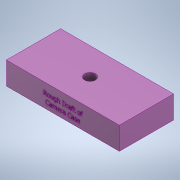
# Autodesk Inventor part: RaspberryPiCameraCase
Saved by Autodesk Inventor 2020.1 (Build 241239000, 239)
## iProperties
Created: 2019-10-02
Part Number: RaspberryPiCameraCase
Material: PC/ABS Plastic
Document SubType Name: Modeling
Designer: steele
Density: 0.357273 g/cm^3
Appearance: Smooth - Purple
Author: steele
Autodesk Inventor part; units mm, degrees
ref_plane "YZ Plane" through (0, 0, 0) normal (1, 0, 0) x (0, 1, 0)
ref_plane "XZ Plane" through (0, 0, 0) normal (0, 1, 0) x (-1, 0, 0)
ref_plane "XY Plane" through (0, 0, 0) normal (0, 0, 1) x (1, 0, 0)
sketch "Sketch1" plane through (0, 0, 0) normal (0, 1, 0) x (-1, 0, 0)
  line L0 (39.6875, 19.05) -> (-39.6875, 19.05)
  line L1 (-39.6875, 19.05) -> (-39.6875, -19.05)
  line L2 (-39.6875, -19.05) -> (39.6875, -19.05)
  line L3 (39.6875, -19.05) -> (39.6875, 19.05)
  line L4 (39.6875, 19.05) -> (-39.6875, -19.05) construction
  line L5 (-39.6875, 19.05) -> (39.6875, -19.05) construction
  point P0 (0, 0)
  dimension "d0" = 79.375
  dimension "d1" = 38.1
  constraints: 12 end point, 2 midpoint, 2 parallel, 1 horizontal, 1 perpendicular
  measures "d0" distance of L1.end L2.end
  measures "d1" distance of L2.end L0.start
extrude "Extrusion1" add sketch "Sketch1" against normal blind 15.875
sketch "Sketch2" plane through (0, 0, 0) normal (0, 1, 0) x (1, 0, 0)
  circle A0 centre (0, 0) radius 3.81
  dimension "d4" = 7.62
  constraints: 1 centre point, 1 coincident
  measures "d4" diameter of A0
extrude "Extrusion2" cut sketch "Sketch2" against normal through all
sketch "Sketch3" plane through (0, -15.875, 0) normal (0, -1, 0) x (1, 0, 0)
  point P0 (0, 0)
sketch "Sketch4" plane through (-39.6875, 0, 19.05) normal (0, 0, 1) x (1, 0, 0)
  line L0 (0, 0) -> (0, -15.875) construction
  line L1 (0, -7.9375) -> (79.375, -7.9375) construction
  line L2 (79.375, 0) -> (79.375, -15.875) construction
  line L3 (28.6181, -7.9375) -> (28.092, -7.9375)
  line L4 (28.092, -7.9375) -> (27.1287, -6.7247)
  line L5 (27.1287, -6.7247) -> (26.6643, -6.7247)
  line L6 (26.6643, -6.7247) -> (26.6643, -7.9375)
  line L7 (26.6643, -7.9375) -> (26.2593, -7.9375)
  line L8 (26.2593, -7.9375) -> (26.2593, -4.8895)
  line L9 (26.2593, -4.8895) -> (27.0447, -4.8895)
  spline S0 degree 2 poles (27.0447, -4.8895) (27.3065, -4.8895) (27.6598, -4.9463) (27.8203, -5.0501) knots 0 0 0 1 2 2 2
  spline S1 degree 2 poles (27.8203, -5.0501) (27.9809, -5.1538) (28.1661, -5.4774) (28.1661, -5.717) knots 0 0 0 1 2 2 2
  spline S2 degree 2 poles (28.1661, -5.717) (28.1661, -6.0504) (27.8252, -6.5024) (27.5338, -6.6111) knots 0 0 0 1 2 2 2
  line L10 (27.5338, -6.6111) -> (28.6181, -7.9375)
  spline S3 degree 2 poles (27.7437, -5.7491) (27.7437, -5.6157) (27.6499, -5.4107) (27.5511, -5.344) knots 0 0 0 1 2 2 2
  spline S4 degree 2 poles (27.5511, -5.344) (27.4646, -5.2872) (27.2349, -5.2402) (27.067, -5.2402) knots 0 0 0 1 2 2 2
  line L11 (27.067, -5.2402) -> (26.6643, -5.2402)
  line L12 (26.6643, -5.2402) -> (26.6643, -6.3863)
  line L13 (26.6643, -6.3863) -> (27.02, -6.3863)
  spline S5 degree 2 poles (27.02, -6.3863) (27.1954, -6.3863) (27.4745, -6.3246) (27.5708, -6.2282) knots 0 0 0 1 2 2 2
  spline S6 degree 2 poles (27.5708, -6.2282) (27.6598, -6.1443) (27.7437, -5.9071) (27.7437, -5.7491) knots 0 0 0 1 2 2 2
  spline S7 degree 2 poles (30.7102, -6.7939) (30.7102, -7.3719) (30.1545, -8.0017) (29.6901, -8.0017) knots 0 0 0 1 2 2 2
  spline S8 degree 2 poles (29.6901, -8.0017) (29.2134, -8.0017) (28.6675, -7.3521) (28.6675, -6.7939) knots 0 0 0 1 2 2 2
  spline S9 degree 2 poles (28.6675, -6.7939) (28.6675, -6.2208) (29.2307, -5.586) (29.6901, -5.586) knots 0 0 0 1 2 2 2
  spline S10 degree 2 poles (29.6901, -5.586) (30.1545, -5.586) (30.7102, -6.2184) (30.7102, -6.7939) knots 0 0 0 1 2 2 2
  spline S11 degree 2 poles (30.3126, -6.7939) (30.3126, -6.3493) (29.989, -5.917) (29.6901, -5.917) knots 0 0 0 1 2 2 2
  spline S12 degree 2 poles (29.6901, -5.917) (29.3912, -5.917) (29.0652, -6.3493) (29.0652, -6.7939) knots 0 0 0 1 2 2 2
  spline S13 degree 2 poles (29.0652, -6.7939) (29.0652, -7.2261) (29.3912, -7.6707) (29.6901, -7.6707) knots 0 0 0 1 2 2 2
  spline S14 degree 2 poles (29.6901, -7.6707) (29.9865, -7.6707) (30.3126, -7.2335) (30.3126, -6.7939) knots 0 0 0 1 2 2 2
  line L14 (32.8838, -7.9375) -> (32.4985, -7.9375)
  line L15 (32.4985, -7.9375) -> (32.4985, -7.6856)
  spline S15 degree 2 poles (32.4985, -7.6856) (32.3207, -7.8412) (32.002, -8.0017) (31.8044, -8.0017) knots 0 0 0 1 2 2 2
  spline S16 degree 2 poles (31.8044, -8.0017) (31.6562, -8.0017) (31.392, -7.9029) (31.2956, -7.7967) knots 0 0 0 1 2 2 2
  spline S17 degree 2 poles (31.2956, -7.7967) (31.1968, -7.6905) (31.0881, -7.3669) (31.0881, -7.1347) knots 0 0 0 1 2 2 2
  line L16 (31.0881, -7.1347) -> (31.0881, -5.6503)
  line L17 (31.0881, -5.6503) -> (31.4735, -5.6503)
  line L18 (31.4735, -5.6503) -> (31.4735, -6.9544)
  spline S18 degree 2 poles (31.4735, -6.9544) (31.4735, -7.1372) (31.5006, -7.3768) (31.5476, -7.4657) knots 0 0 0 1 2 2 2
  spline S19 degree 2 poles (31.5476, -7.4657) (31.5945, -7.5546) (31.755, -7.6362) (31.9057, -7.6362) knots 0 0 0 1 2 2 2
  spline S20 degree 2 poles (31.9057, -7.6362) (32.0465, -7.6362) (32.3651, -7.4756) (32.4985, -7.3595) knots 0 0 0 1 2 2 2
  line L19 (32.4985, -7.3595) -> (32.4985, -5.6503)
  line L20 (32.4985, -5.6503) -> (32.8838, -5.6503)
  line L21 (32.8838, -5.6503) -> (32.8838, -7.9375)
  spline S21 degree 2 poles (33.5236, -8.3031) (33.5631, -8.3204) (33.7138, -8.3747) (33.8101, -8.3969) knots 0 0 0 1 2 2 2
  spline S22 degree 2 poles (33.8101, -8.3969) (33.9163, -8.4241) (34.0966, -8.4562) (34.2028, -8.4562) knots 0 0 0 1 2 2 2
  spline S23 degree 2 poles (34.2028, -8.4562) (34.3807, -8.4562) (34.6277, -8.3623) (34.6968, -8.2784) knots 0 0 0 1 2 2 2
  spline S24 degree 2 poles (34.6968, -8.2784) (34.7635, -8.1944) (34.8154, -7.9746) (34.8154, -7.8338) knots 0 0 0 1 2 2 2
  line L22 (34.8154, -7.8338) -> (34.8154, -7.6337)
  spline S25 degree 2 poles (34.8154, -7.6337) (34.6598, -7.7695) (34.3609, -7.898) (34.1361, -7.898) knots 0 0 0 1 2 2 2
  spline S26 degree 2 poles (34.1361, -7.898) (33.7459, -7.898) (33.284, -7.3175) (33.284, -6.7717) knots 0 0 0 1 2 2 2
  spline S27 degree 2 poles (33.284, -6.7717) (33.284, -6.4876) (33.4445, -6.0479) (33.5779, -5.8923) knots 0 0 0 1 2 2 2
  spline S28 degree 2 poles (33.5779, -5.8923) (33.7064, -5.7466) (34.0596, -5.586) (34.2473, -5.586) knots 0 0 0 1 2 2 2
  spline S29 degree 2 poles (34.2473, -5.586) (34.4251, -5.586) (34.6845, -5.67) (34.8154, -5.7466) knots 0 0 0 1 2 2 2
  line L23 (34.8154, -5.7466) -> (34.8376, -5.6503)
  line L24 (34.8376, -5.6503) -> (35.2007, -5.6503)
  line L25 (35.2007, -5.6503) -> (35.2007, -7.6757)
  spline S30 degree 2 poles (35.2007, -7.6757) (35.2007, -8.2586) (34.6944, -8.802) (34.1732, -8.802) knots 0 0 0 1 2 2 2
  spline S31 degree 2 poles (34.1732, -8.802) (34.0052, -8.802) (33.6545, -8.7477) (33.5038, -8.7032) knots 0 0 0 1 2 2 2
  line L26 (33.5038, -8.7032) -> (33.5038, -8.3031)
  line L27 (33.5038, -8.3031) -> (33.5236, -8.3031)
  line L28 (34.8154, -7.3175) -> (34.8154, -6.0603)
  spline S32 degree 2 poles (34.8154, -6.0603) (34.6721, -5.9911) (34.4301, -5.9318) (34.309, -5.9318) knots 0 0 0 1 2 2 2
  spline S33 degree 2 poles (34.309, -5.9318) (34.0176, -5.9318) (33.6817, -6.3616) (33.6817, -6.7642) knots 0 0 0 1 2 2 2
  spline S34 degree 2 poles (33.6817, -6.7642) (33.6817, -7.1446) (33.9361, -7.5423) (34.2226, -7.5423) knots 0 0 0 1 2 2 2
  spline S35 degree 2 poles (34.2226, -7.5423) (34.3733, -7.5423) (34.6894, -7.4237) (34.8154, -7.3175) knots 0 0 0 1 2 2 2
  line L29 (37.5546, -7.9375) -> (37.1693, -7.9375)
  line L30 (37.1693, -7.9375) -> (37.1693, -6.6333)
  spline S36 degree 2 poles (37.1693, -6.6333) (37.1693, -6.4753) (37.1397, -6.2035) (37.0952, -6.122) knots 0 0 0 1 2 2 2
  spline S37 degree 2 poles (37.0952, -6.122) (37.0483, -6.0356) (36.8803, -5.9516) (36.7371, -5.9516) knots 0 0 0 1 2 2 2
  spline S38 degree 2 poles (36.7371, -5.9516) (36.5938, -5.9516) (36.29, -6.1047) (36.1443, -6.2282) knots 0 0 0 1 2 2 2
  line L31 (36.1443, -6.2282) -> (36.1443, -7.9375)
  line L32 (36.1443, -7.9375) -> (35.7589, -7.9375)
  line L33 (35.7589, -7.9375) -> (35.7589, -4.7536)
  line L34 (35.7589, -4.7536) -> (36.1443, -4.7536)
  line L35 (36.1443, -4.7536) -> (36.1443, -5.9047)
  spline S39 degree 2 poles (36.1443, -5.9047) (36.3172, -5.7491) (36.6506, -5.586) (36.8383, -5.586) knots 0 0 0 1 2 2 2
  spline S40 degree 2 poles (36.8383, -5.586) (37.1743, -5.586) (37.5546, -6.0306) (37.5546, -6.453) knots 0 0 0 1 2 2 2
  line L36 (37.5546, -6.453) -> (37.5546, -7.9375)
  spline S41 degree 2 poles (41.8376, -6.416) (41.8376, -6.8334) (41.4993, -7.5052) (41.2152, -7.693) knots 0 0 0 1 2 2 2
  spline S42 degree 2 poles (41.2152, -7.693) (40.983, -7.8387) (40.5063, -7.9375) (40.1358, -7.9375) knots 0 0 0 1 2 2 2
  line L37 (40.1358, -7.9375) -> (39.4343, -7.9375)
  line L38 (39.4343, -7.9375) -> (39.4343, -4.8895)
  line L39 (39.4343, -4.8895) -> (40.1284, -4.8895)
  spline S43 degree 2 poles (40.1284, -4.8895) (40.5582, -4.8895) (41.0472, -5.0179) (41.2201, -5.1316) knots 0 0 0 1 2 2 2
  spline S44 degree 2 poles (41.2201, -5.1316) (41.5141, -5.3267) (41.8376, -5.9714) (41.8376, -6.416) knots 0 0 0 1 2 2 2
  spline S45 degree 2 poles (41.4153, -6.411) (41.4153, -6.0603) (41.1831, -5.5638) (40.9534, -5.423) knots 0 0 0 1 2 2 2
  spline S46 degree 2 poles (40.9534, -5.423) (40.7904, -5.3267) (40.4223, -5.2402) (40.1482, -5.2402) knots 0 0 0 1 2 2 2
  line L40 (40.1482, -5.2402) -> (39.8394, -5.2402)
  line L41 (39.8394, -5.2402) -> (39.8394, -7.5868)
  line L42 (39.8394, -7.5868) -> (40.1482, -7.5868)
  spline S47 degree 2 poles (40.1482, -7.5868) (40.4174, -7.5868) (40.8249, -7.5003) (40.9904, -7.3842) knots 0 0 0 1 2 2 2
  spline S48 degree 2 poles (40.9904, -7.3842) (41.2029, -7.241) (41.4153, -6.7667) (41.4153, -6.411) knots 0 0 0 1 2 2 2
  line L43 (43.4604, -6.0628) -> (43.4407, -6.0628)
  spline S49 degree 2 poles (43.4407, -6.0628) (43.3962, -6.0504) (43.2999, -6.0455) (43.2332, -6.0455) knots 0 0 0 1 2 2 2
  spline S50 degree 2 poles (43.2332, -6.0455) (43.0776, -6.0455) (42.7713, -6.1813) (42.633, -6.3147) knots 0 0 0 1 2 2 2
  line L44 (42.633, -6.3147) -> (42.633, -7.9375)
  line L45 (42.633, -7.9375) -> (42.2477, -7.9375)
  line L46 (42.2477, -7.9375) -> (42.2477, -5.6503)
  line L47 (42.2477, -5.6503) -> (42.633, -5.6503)
  line L48 (42.633, -5.6503) -> (42.633, -5.9911)
  spline S51 degree 2 poles (42.633, -5.9911) (42.8429, -5.8034) (43.1566, -5.6503) (43.3048, -5.6503) knots 0 0 0 1 2 2 2
  spline S52 degree 2 poles (43.3048, -5.6503) (43.3641, -5.6503) (43.4234, -5.6552) (43.4604, -5.6626) knots 0 0 0 1 2 2 2
  line L49 (43.4604, -5.6626) -> (43.4604, -6.0628)
  spline S53 degree 2 poles (45.0338, -7.6954) (44.9869, -7.73) (44.8288, -7.8535) (44.7547, -7.8906) knots 0 0 0 1 2 2 2
  spline S54 degree 2 poles (44.7547, -7.8906) (44.6535, -7.9449) (44.4633, -8.0017) (44.2904, -8.0017) knots 0 0 0 1 2 2 2
  spline S55 degree 2 poles (44.2904, -8.0017) (44.1496, -8.0017) (43.8952, -7.8955) (43.7988, -7.7992) knots 0 0 0 1 2 2 2
  spline S56 degree 2 poles (43.7988, -7.7992) (43.7075, -7.7053) (43.5963, -7.4287) (43.5963, -7.2755) knots 0 0 0 1 2 2 2
  spline S57 degree 2 poles (43.5963, -7.2755) (43.5963, -7.0384) (43.7964, -6.7025) (44.0137, -6.6062) knots 0 0 0 1 2 2 2
  spline S58 degree 2 poles (44.0137, -6.6062) (44.2064, -6.5172) (44.73, -6.4506) (45.0338, -6.4333) knots 0 0 0 1 2 2 2
  line L50 (45.0338, -6.4333) -> (45.0338, -6.3592)
  spline S59 degree 2 poles (45.0338, -6.3592) (45.0338, -6.2258) (44.9523, -6.0603) (44.8782, -6.0134) knots 0 0 0 1 2 2 2
  spline S60 degree 2 poles (44.8782, -6.0134) (44.8041, -5.9664) (44.5917, -5.9368) (44.4781, -5.9368) knots 0 0 0 1 2 2 2
  spline S61 degree 2 poles (44.4781, -5.9368) (44.3447, -5.9368) (43.9841, -6.0158) (43.8038, -6.0924) knots 0 0 0 1 2 2 2
  line L51 (43.8038, -6.0924) -> (43.7816, -6.0924)
  line L52 (43.7816, -6.0924) -> (43.7816, -5.6997)
  spline S62 degree 2 poles (43.7816, -5.6997) (43.8878, -5.67) (44.2854, -5.5959) (44.4806, -5.5959) knots 0 0 0 1 2 2 2
  spline S63 degree 2 poles (44.4806, -5.5959) (44.7177, -5.5959) (45.0413, -5.67) (45.1697, -5.7664) knots 0 0 0 1 2 2 2
  spline S64 degree 2 poles (45.1697, -5.7664) (45.2957, -5.8602) (45.4192, -6.1591) (45.4192, -6.374) knots 0 0 0 1 2 2 2
  line L53 (45.4192, -6.374) -> (45.4192, -7.9375)
  line L54 (45.4192, -7.9375) -> (45.0338, -7.9375)
  line L55 (45.0338, -7.9375) -> (45.0338, -7.6954)
  line L56 (45.0338, -7.3743) -> (45.0338, -6.7395)
  spline S65 degree 2 poles (45.0338, -6.7395) (44.8955, -6.7519) (44.4781, -6.7939) (44.3472, -6.8334) knots 0 0 0 1 2 2 2
  spline S66 degree 2 poles (44.3472, -6.8334) (44.194, -6.8803) (43.994, -7.0755) (43.994, -7.2484) knots 0 0 0 1 2 2 2
  spline S67 degree 2 poles (43.994, -7.2484) (43.994, -7.446) (44.2163, -7.646) (44.4287, -7.646) knots 0 0 0 1 2 2 2
  spline S68 degree 2 poles (44.4287, -7.646) (44.609, -7.646) (44.9054, -7.4904) (45.0338, -7.3743) knots 0 0 0 1 2 2 2
  line L57 (47.163, -5.1242) -> (47.1432, -5.1242)
  spline S69 degree 2 poles (47.1432, -5.1242) (47.0914, -5.1044) (46.8987, -5.0698) (46.8221, -5.0698) knots 0 0 0 1 2 2 2
  spline S70 degree 2 poles (46.8221, -5.0698) (46.5801, -5.0698) (46.3726, -5.2872) (46.3726, -5.5737) knots 0 0 0 1 2 2 2
  line L58 (46.3726, -5.5737) -> (46.3726, -5.6503)
  line L59 (46.3726, -5.6503) -> (47.0099, -5.6503)
  line L60 (47.0099, -5.6503) -> (47.0099, -5.9689)
  line L61 (47.0099, -5.9689) -> (46.3849, -5.9689)
  line L62 (46.3849, -5.9689) -> (46.3849, -7.9375)
  line L63 (46.3849, -7.9375) -> (45.9996, -7.9375)
  line L64 (45.9996, -7.9375) -> (45.9996, -5.9689)
  line L65 (45.9996, -5.9689) -> (45.7403, -5.9689)
  line L66 (45.7403, -5.9689) -> (45.7403, -5.6503)
  line L67 (45.7403, -5.6503) -> (45.9996, -5.6503)
  line L68 (45.9996, -5.6503) -> (45.9996, -5.5737)
  spline S71 degree 2 poles (45.9996, -5.5737) (45.9996, -5.1637) (46.3973, -4.7339) (46.7678, -4.7339) knots 0 0 0 1 2 2 2
  spline S72 degree 2 poles (46.7678, -4.7339) (46.874, -4.7339) (47.079, -4.7561) (47.163, -4.7709) knots 0 0 0 1 2 2 2
  line L69 (47.163, -4.7709) -> (47.163, -5.1242)
  spline S73 degree 2 poles (48.0744, -7.982) (47.7607, -7.982) (47.4075, -7.6238) (47.4075, -7.236) knots 0 0 0 1 2 2 2
  line L70 (47.4075, -7.236) -> (47.4075, -5.9689)
  line L71 (47.4075, -5.9689) -> (47.1482, -5.9689)
  line L72 (47.1482, -5.9689) -> (47.1482, -5.6503)
  line L73 (47.1482, -5.6503) -> (47.4075, -5.6503)
  line L74 (47.4075, -5.6503) -> (47.4075, -4.9932)
  line L75 (47.4075, -4.9932) -> (47.7929, -4.9932)
  line L76 (47.7929, -4.9932) -> (47.7929, -5.6503)
  line L77 (47.7929, -5.6503) -> (48.5018, -5.6503)
  line L78 (48.5018, -5.6503) -> (48.5018, -5.9689)
  line L79 (48.5018, -5.9689) -> (47.7929, -5.9689)
  line L80 (47.7929, -5.9689) -> (47.7929, -7.0582)
  spline S74 degree 2 poles (47.7929, -7.0582) (47.7929, -7.2311) (47.8052, -7.4213) (47.8472, -7.5028) knots 0 0 0 1 2 2 2
  spline S75 degree 2 poles (47.8472, -7.5028) (47.8818, -7.5744) (48.0374, -7.646) (48.1708, -7.646) knots 0 0 0 1 2 2 2
  spline S76 degree 2 poles (48.1708, -7.646) (48.2646, -7.646) (48.44, -7.5892) (48.4795, -7.5719) knots 0 0 0 1 2 2 2
  line L81 (48.4795, -7.5719) -> (48.5018, -7.5719)
  line L82 (48.5018, -7.5719) -> (48.5018, -7.9177)
  spline S77 degree 2 poles (48.5018, -7.9177) (48.3931, -7.9474) (48.1708, -7.982) (48.0744, -7.982) knots 0 0 0 1 2 2 2
  spline S78 degree 2 poles (51.9746, -6.7939) (51.9746, -7.3719) (51.4188, -8.0017) (50.9545, -8.0017) knots 0 0 0 1 2 2 2
  spline S79 degree 2 poles (50.9545, -8.0017) (50.4778, -8.0017) (49.9319, -7.3521) (49.9319, -6.7939) knots 0 0 0 1 2 2 2
  spline S80 degree 2 poles (49.9319, -6.7939) (49.9319, -6.2208) (50.4951, -5.586) (50.9545, -5.586) knots 0 0 0 1 2 2 2
  spline S81 degree 2 poles (50.9545, -5.586) (51.4188, -5.586) (51.9746, -6.2184) (51.9746, -6.7939) knots 0 0 0 1 2 2 2
  spline S82 degree 2 poles (51.5769, -6.7939) (51.5769, -6.3493) (51.2534, -5.917) (50.9545, -5.917) knots 0 0 0 1 2 2 2
  spline S83 degree 2 poles (50.9545, -5.917) (50.6556, -5.917) (50.3296, -6.3493) (50.3296, -6.7939) knots 0 0 0 1 2 2 2
  spline S84 degree 2 poles (50.3296, -6.7939) (50.3296, -7.2261) (50.6556, -7.6707) (50.9545, -7.6707) knots 0 0 0 1 2 2 2
  spline S85 degree 2 poles (50.9545, -7.6707) (51.2509, -7.6707) (51.5769, -7.2335) (51.5769, -6.7939) knots 0 0 0 1 2 2 2
  line L83 (53.5727, -5.1242) -> (53.5529, -5.1242)
  spline S86 degree 2 poles (53.5529, -5.1242) (53.5011, -5.1044) (53.3084, -5.0698) (53.2318, -5.0698) knots 0 0 0 1 2 2 2
  spline S87 degree 2 poles (53.2318, -5.0698) (52.9898, -5.0698) (52.7823, -5.2872) (52.7823, -5.5737) knots 0 0 0 1 2 2 2
  line L84 (52.7823, -5.5737) -> (52.7823, -5.6503)
  line L85 (52.7823, -5.6503) -> (53.4196, -5.6503)
  line L86 (53.4196, -5.6503) -> (53.4196, -5.9689)
  line L87 (53.4196, -5.9689) -> (52.7946, -5.9689)
  line L88 (52.7946, -5.9689) -> (52.7946, -7.9375)
  line L89 (52.7946, -7.9375) -> (52.4093, -7.9375)
  line L90 (52.4093, -7.9375) -> (52.4093, -5.9689)
  line L91 (52.4093, -5.9689) -> (52.15, -5.9689)
  line L92 (52.15, -5.9689) -> (52.15, -5.6503)
  line L93 (52.15, -5.6503) -> (52.4093, -5.6503)
  line L94 (52.4093, -5.6503) -> (52.4093, -5.5737)
  spline S88 degree 2 poles (52.4093, -5.5737) (52.4093, -5.1637) (52.807, -4.7339) (53.1775, -4.7339) knots 0 0 0 1 2 2 2
  spline S89 degree 2 poles (53.1775, -4.7339) (53.2837, -4.7339) (53.4887, -4.7561) (53.5727, -4.7709) knots 0 0 0 1 2 2 2
  line L95 (53.5727, -4.7709) -> (53.5727, -5.1242)
  spline S90 degree 2 poles (29.0578, -13.0153) (28.7614, -13.0153) (28.26, -12.8152) (28.0772, -12.6152) knots 0 0 0 1 2 2 2
  spline S91 degree 2 poles (28.0772, -12.6152) (27.8944, -12.4176) (27.6943, -11.8248) (27.6943, -11.4394) knots 0 0 0 1 2 2 2
  spline S92 degree 2 poles (27.6943, -11.4394) (27.6943, -11.0566) (27.8895, -10.4885) (28.0747, -10.2785) knots 0 0 0 1 2 2 2
  spline S93 degree 2 poles (28.0747, -10.2785) (28.2575, -10.0735) (28.7564, -9.8586) (29.0652, -9.8586) knots 0 0 0 1 2 2 2
  spline S94 degree 2 poles (29.0652, -9.8586) (29.2183, -9.8586) (29.4876, -9.9031) (29.6012, -9.9377) knots 0 0 0 1 2 2 2
  spline S95 degree 2 poles (29.6012, -9.9377) (29.7, -9.9698) (29.905, -10.0612) (30.0063, -10.1155) knots 0 0 0 1 2 2 2
  line L96 (30.0063, -10.1155) -> (30.0063, -10.6046)
  line L97 (30.0063, -10.6046) -> (29.9742, -10.6046)
  spline S96 degree 2 poles (29.9742, -10.6046) (29.9198, -10.5552) (29.7519, -10.4168) (29.6308, -10.3502) knots 0 0 0 1 2 2 2
  spline S97 degree 2 poles (29.6308, -10.3502) (29.5147, -10.2859) (29.2406, -10.2044) (29.0627, -10.2044) knots 0 0 0 1 2 2 2
  spline S98 degree 2 poles (29.0627, -10.2044) (28.8676, -10.2044) (28.5193, -10.365) (28.3884, -10.5181) knots 0 0 0 1 2 2 2
  spline S99 degree 2 poles (28.3884, -10.5181) (28.26, -10.6737) (28.1167, -11.1455) (28.1167, -11.4394) knots 0 0 0 1 2 2 2
  spline S100 degree 2 poles (28.1167, -11.4394) (28.1167, -11.7531) (28.2674, -12.2051) (28.3983, -12.3607) knots 0 0 0 1 2 2 2
  spline S101 degree 2 poles (28.3983, -12.3607) (28.5267, -12.5114) (28.8701, -12.6646) (29.0627, -12.6646) knots 0 0 0 1 2 2 2
  spline S102 degree 2 poles (29.0627, -12.6646) (29.2381, -12.6646) (29.537, -12.5781) (29.6531, -12.5139) knots 0 0 0 1 2 2 2
  spline S103 degree 2 poles (29.6531, -12.5139) (29.7642, -12.4497) (29.9297, -12.3163) (29.9766, -12.2694) knots 0 0 0 1 2 2 2
  line L98 (29.9766, -12.2694) -> (30.0063, -12.2694)
  line L99 (30.0063, -12.2694) -> (30.0063, -12.7535)
  spline S104 degree 2 poles (30.0063, -12.7535) (29.905, -12.8004) (29.7272, -12.8869) (29.6012, -12.9264) knots 0 0 0 1 2 2 2
  spline S105 degree 2 poles (29.6012, -12.9264) (29.4678, -12.9708) (29.2406, -13.0153) (29.0578, -13.0153) knots 0 0 0 1 2 2 2
  spline S106 degree 2 poles (31.6291, -12.7189) (31.5821, -12.7535) (31.4241, -12.877) (31.35, -12.914) knots 0 0 0 1 2 2 2
  spline S107 degree 2 poles (31.35, -12.914) (31.2487, -12.9684) (31.0585, -13.0252) (30.8856, -13.0252) knots 0 0 0 1 2 2 2
  spline S108 degree 2 poles (30.8856, -13.0252) (30.7448, -13.0252) (30.4904, -12.919) (30.3941, -12.8226) knots 0 0 0 1 2 2 2
  spline S109 degree 2 poles (30.3941, -12.8226) (30.3027, -12.7288) (30.1915, -12.4521) (30.1915, -12.299) knots 0 0 0 1 2 2 2
  spline S110 degree 2 poles (30.1915, -12.299) (30.1915, -12.0619) (30.3916, -11.726) (30.609, -11.6296) knots 0 0 0 1 2 2 2
  spline S111 degree 2 poles (30.609, -11.6296) (30.8016, -11.5407) (31.3253, -11.474) (31.6291, -11.4567) knots 0 0 0 1 2 2 2
  line L100 (31.6291, -11.4567) -> (31.6291, -11.3826)
  spline S112 degree 2 poles (31.6291, -11.3826) (31.6291, -11.2492) (31.5476, -11.0838) (31.4735, -11.0368) knots 0 0 0 1 2 2 2
  spline S113 degree 2 poles (31.4735, -11.0368) (31.3994, -10.9899) (31.1869, -10.9602) (31.0733, -10.9602) knots 0 0 0 1 2 2 2
  spline S114 degree 2 poles (31.0733, -10.9602) (30.9399, -10.9602) (30.5793, -11.0393) (30.399, -11.1159) knots 0 0 0 1 2 2 2
  line L101 (30.399, -11.1159) -> (30.3768, -11.1159)
  line L102 (30.3768, -11.1159) -> (30.3768, -10.7231)
  spline S115 degree 2 poles (30.3768, -10.7231) (30.483, -10.6935) (30.8807, -10.6194) (31.0758, -10.6194) knots 0 0 0 1 2 2 2
  spline S116 degree 2 poles (31.0758, -10.6194) (31.3129, -10.6194) (31.6365, -10.6935) (31.7649, -10.7898) knots 0 0 0 1 2 2 2
  spline S117 degree 2 poles (31.7649, -10.7898) (31.8909, -10.8837) (32.0144, -11.1826) (32.0144, -11.3974) knots 0 0 0 1 2 2 2
  line L103 (32.0144, -11.3974) -> (32.0144, -12.961)
  line L104 (32.0144, -12.961) -> (31.6291, -12.961)
  line L105 (31.6291, -12.961) -> (31.6291, -12.7189)
  line L106 (31.6291, -12.3978) -> (31.6291, -11.763)
  spline S118 degree 2 poles (31.6291, -11.763) (31.4908, -11.7754) (31.0733, -11.8173) (30.9424, -11.8569) knots 0 0 0 1 2 2 2
  spline S119 degree 2 poles (30.9424, -11.8569) (30.7893, -11.9038) (30.5892, -12.0989) (30.5892, -12.2718) knots 0 0 0 1 2 2 2
  spline S120 degree 2 poles (30.5892, -12.2718) (30.5892, -12.4694) (30.8115, -12.6695) (31.0239, -12.6695) knots 0 0 0 1 2 2 2
  spline S121 degree 2 poles (31.0239, -12.6695) (31.2042, -12.6695) (31.5006, -12.5139) (31.6291, -12.3978) knots 0 0 0 1 2 2 2
  line L107 (35.1488, -12.961) -> (35.1488, -11.637)
  spline S122 degree 2 poles (35.1488, -11.637) (35.1488, -11.479) (35.1241, -11.2097) (35.0846, -11.1356) knots 0 0 0 1 2 2 2
  spline S123 degree 2 poles (35.0846, -11.1356) (35.0451, -11.0541) (34.8944, -10.9751) (34.7635, -10.9751) knots 0 0 0 1 2 2 2
  spline S124 degree 2 poles (34.7635, -10.9751) (34.645, -10.9751) (34.3733, -11.1208) (34.23, -11.2591) knots 0 0 0 1 2 2 2
  spline S125 degree 2 poles (34.23, -11.2591) (34.2325, -11.2937) (34.2374, -11.39) (34.2374, -11.4543) knots 0 0 0 1 2 2 2
  line L108 (34.2374, -11.4543) -> (34.2374, -12.961)
  line L109 (34.2374, -12.961) -> (33.8521, -12.961)
  line L110 (33.8521, -12.961) -> (33.8521, -11.637)
  spline S126 degree 2 poles (33.8521, -11.637) (33.8521, -11.479) (33.8274, -11.2097) (33.7879, -11.1356) knots 0 0 0 1 2 2 2
  spline S127 degree 2 poles (33.7879, -11.1356) (33.7483, -11.0541) (33.5977, -10.9751) (33.4668, -10.9751) knots 0 0 0 1 2 2 2
  spline S128 degree 2 poles (33.4668, -10.9751) (33.3433, -10.9751) (33.0691, -11.1307) (32.9407, -11.2517) knots 0 0 0 1 2 2 2
  line L111 (32.9407, -11.2517) -> (32.9407, -12.961)
  line L112 (32.9407, -12.961) -> (32.5553, -12.961)
  line L113 (32.5553, -12.961) -> (32.5553, -10.6737)
  line L114 (32.5553, -10.6737) -> (32.9407, -10.6737)
  line L115 (32.9407, -10.6737) -> (32.9407, -10.9257)
  spline S129 degree 2 poles (32.9407, -10.9257) (33.0913, -10.775) (33.3877, -10.6095) (33.5656, -10.6095) knots 0 0 0 1 2 2 2
  spline S130 degree 2 poles (33.5656, -10.6095) (33.7681, -10.6095) (34.0818, -10.7948) (34.1633, -11.0047) knots 0 0 0 1 2 2 2
  spline S131 degree 2 poles (34.1633, -11.0047) (34.3387, -10.8096) (34.6697, -10.6095) (34.8623, -10.6095) knots 0 0 0 1 2 2 2
  spline S132 degree 2 poles (34.8623, -10.6095) (35.0105, -10.6095) (35.2526, -10.7009) (35.3415, -10.8046) knots 0 0 0 1 2 2 2
  spline S133 degree 2 poles (35.3415, -10.8046) (35.4329, -10.9084) (35.5342, -11.2196) (35.5342, -11.4543) knots 0 0 0 1 2 2 2
  line L116 (35.5342, -11.4543) -> (35.5342, -12.961)
  line L117 (35.5342, -12.961) -> (35.1488, -12.961)
  spline S134 degree 2 poles (37.068, -13.0128) (36.5197, -13.0128) (35.917, -12.3978) (35.917, -11.8297) knots 0 0 0 1 2 2 2
  spline S135 degree 2 poles (35.917, -11.8297) (35.917, -11.2715) (36.5024, -10.6095) (36.9742, -10.6095) knots 0 0 0 1 2 2 2
  spline S136 degree 2 poles (36.9742, -10.6095) (37.1866, -10.6095) (37.5151, -10.733) (37.6362, -10.8639) knots 0 0 0 1 2 2 2
  spline S137 degree 2 poles (37.6362, -10.8639) (37.7597, -10.9948) (37.8906, -11.3727) (37.8906, -11.6469) knots 0 0 0 1 2 2 2
  line L118 (37.8906, -11.6469) -> (37.8906, -11.8569)
  line L119 (37.8906, -11.8569) -> (36.3073, -11.8569)
  spline S138 degree 2 poles (36.3073, -11.8569) (36.3073, -12.2545) (36.7074, -12.6769) (37.0631, -12.6769) knots 0 0 0 1 2 2 2
  spline S139 degree 2 poles (37.0631, -12.6769) (37.1891, -12.6769) (37.4336, -12.6201) (37.5324, -12.5756) knots 0 0 0 1 2 2 2
  spline S140 degree 2 poles (37.5324, -12.5756) (37.6362, -12.5262) (37.7794, -12.4398) (37.8263, -12.4003) knots 0 0 0 1 2 2 2
  line L120 (37.8263, -12.4003) -> (37.8486, -12.4003)
  line L121 (37.8486, -12.4003) -> (37.8486, -12.8202)
  spline S141 degree 2 poles (37.8486, -12.8202) (37.7819, -12.8473) (37.5793, -12.9264) (37.5003, -12.9486) knots 0 0 0 1 2 2 2
  spline S142 degree 2 poles (37.5003, -12.9486) (37.3891, -12.9807) (37.2064, -13.0128) (37.068, -13.0128) knots 0 0 0 1 2 2 2
  spline S143 degree 2 poles (37.5151, -11.5629) (37.5102, -11.4073) (37.446, -11.1801) (37.3842, -11.1035) knots 0 0 0 1 2 2 2
  spline S144 degree 2 poles (37.3842, -11.1035) (37.3175, -11.0171) (37.1076, -10.9257) (36.952, -10.9257) knots 0 0 0 1 2 2 2
  spline S145 degree 2 poles (36.952, -10.9257) (36.7988, -10.9257) (36.5839, -11.0171) (36.495, -11.106) knots 0 0 0 1 2 2 2
  spline S146 degree 2 poles (36.495, -11.106) (36.4086, -11.1974) (36.3196, -11.4172) (36.3073, -11.5629) knots 0 0 0 1 2 2 2
  line L122 (36.3073, -11.5629) -> (37.5151, -11.5629)
  line L123 (39.4936, -11.0862) -> (39.4738, -11.0862)
  spline S147 degree 2 poles (39.4738, -11.0862) (39.4294, -11.0739) (39.3331, -11.0689) (39.2664, -11.0689) knots 0 0 0 1 2 2 2
  spline S148 degree 2 poles (39.2664, -11.0689) (39.1108, -11.0689) (38.8045, -11.2048) (38.6661, -11.3382) knots 0 0 0 1 2 2 2
  line L124 (38.6661, -11.3382) -> (38.6661, -12.961)
  line L125 (38.6661, -12.961) -> (38.2808, -12.961)
  line L126 (38.2808, -12.961) -> (38.2808, -10.6737)
  line L127 (38.2808, -10.6737) -> (38.6661, -10.6737)
  line L128 (38.6661, -10.6737) -> (38.6661, -11.0146)
  spline S149 degree 2 poles (38.6661, -11.0146) (38.8761, -10.8269) (39.1898, -10.6737) (39.338, -10.6737) knots 0 0 0 1 2 2 2
  spline S150 degree 2 poles (39.338, -10.6737) (39.3973, -10.6737) (39.4566, -10.6787) (39.4936, -10.6861) knots 0 0 0 1 2 2 2
  line L129 (39.4936, -10.6861) -> (39.4936, -11.0862)
  spline S151 degree 2 poles (41.067, -12.7189) (41.0201, -12.7535) (40.862, -12.877) (40.7879, -12.914) knots 0 0 0 1 2 2 2
  spline S152 degree 2 poles (40.7879, -12.914) (40.6866, -12.9684) (40.4964, -13.0252) (40.3235, -13.0252) knots 0 0 0 1 2 2 2
  spline S153 degree 2 poles (40.3235, -13.0252) (40.1827, -13.0252) (39.9283, -12.919) (39.832, -12.8226) knots 0 0 0 1 2 2 2
  spline S154 degree 2 poles (39.832, -12.8226) (39.7406, -12.7288) (39.6295, -12.4521) (39.6295, -12.299) knots 0 0 0 1 2 2 2
  spline S155 degree 2 poles (39.6295, -12.299) (39.6295, -12.0619) (39.8295, -11.726) (40.0469, -11.6296) knots 0 0 0 1 2 2 2
  spline S156 degree 2 poles (40.0469, -11.6296) (40.2395, -11.5407) (40.7632, -11.474) (41.067, -11.4567) knots 0 0 0 1 2 2 2
  line L130 (41.067, -11.4567) -> (41.067, -11.3826)
  spline S157 degree 2 poles (41.067, -11.3826) (41.067, -11.2492) (40.9855, -11.0838) (40.9114, -11.0368) knots 0 0 0 1 2 2 2
  spline S158 degree 2 poles (40.9114, -11.0368) (40.8373, -10.9899) (40.6249, -10.9602) (40.5113, -10.9602) knots 0 0 0 1 2 2 2
  spline S159 degree 2 poles (40.5113, -10.9602) (40.3779, -10.9602) (40.0172, -11.0393) (39.8369, -11.1159) knots 0 0 0 1 2 2 2
  line L131 (39.8369, -11.1159) -> (39.8147, -11.1159)
  line L132 (39.8147, -11.1159) -> (39.8147, -10.7231)
  spline S160 degree 2 poles (39.8147, -10.7231) (39.9209, -10.6935) (40.3186, -10.6194) (40.5137, -10.6194) knots 0 0 0 1 2 2 2
  spline S161 degree 2 poles (40.5137, -10.6194) (40.7508, -10.6194) (41.0744, -10.6935) (41.2029, -10.7898) knots 0 0 0 1 2 2 2
  spline S162 degree 2 poles (41.2029, -10.7898) (41.3288, -10.8837) (41.4523, -11.1826) (41.4523, -11.3974) knots 0 0 0 1 2 2 2
  line L133 (41.4523, -11.3974) -> (41.4523, -12.961)
  line L134 (41.4523, -12.961) -> (41.067, -12.961)
  line L135 (41.067, -12.961) -> (41.067, -12.7189)
  line L136 (41.067, -12.3978) -> (41.067, -11.763)
  spline S163 degree 2 poles (41.067, -11.763) (40.9287, -11.7754) (40.5113, -11.8173) (40.3803, -11.8569) knots 0 0 0 1 2 2 2
  spline S164 degree 2 poles (40.3803, -11.8569) (40.2272, -11.9038) (40.0271, -12.0989) (40.0271, -12.2718) knots 0 0 0 1 2 2 2
  spline S165 degree 2 poles (40.0271, -12.2718) (40.0271, -12.4694) (40.2494, -12.6695) (40.4618, -12.6695) knots 0 0 0 1 2 2 2
  spline S166 degree 2 poles (40.4618, -12.6695) (40.6422, -12.6695) (40.9386, -12.5139) (41.067, -12.3978) knots 0 0 0 1 2 2 2
  spline S167 degree 2 poles (44.5226, -13.0153) (44.2262, -13.0153) (43.7247, -12.8152) (43.542, -12.6152) knots 0 0 0 1 2 2 2
  spline S168 degree 2 poles (43.542, -12.6152) (43.3592, -12.4176) (43.1591, -11.8248) (43.1591, -11.4394) knots 0 0 0 1 2 2 2
  spline S169 degree 2 poles (43.1591, -11.4394) (43.1591, -11.0566) (43.3542, -10.4885) (43.5395, -10.2785) knots 0 0 0 1 2 2 2
  spline S170 degree 2 poles (43.5395, -10.2785) (43.7223, -10.0735) (44.2212, -9.8586) (44.53, -9.8586) knots 0 0 0 1 2 2 2
  spline S171 degree 2 poles (44.53, -9.8586) (44.6831, -9.8586) (44.9523, -9.9031) (45.066, -9.9377) knots 0 0 0 1 2 2 2
  spline S172 degree 2 poles (45.066, -9.9377) (45.1648, -9.9698) (45.3698, -10.0612) (45.471, -10.1155) knots 0 0 0 1 2 2 2
  line L137 (45.471, -10.1155) -> (45.471, -10.6046)
  line L138 (45.471, -10.6046) -> (45.4389, -10.6046)
  spline S173 degree 2 poles (45.4389, -10.6046) (45.3846, -10.5552) (45.2166, -10.4168) (45.0956, -10.3502) knots 0 0 0 1 2 2 2
  spline S174 degree 2 poles (45.0956, -10.3502) (44.9795, -10.2859) (44.7053, -10.2044) (44.5275, -10.2044) knots 0 0 0 1 2 2 2
  spline S175 degree 2 poles (44.5275, -10.2044) (44.3324, -10.2044) (43.9841, -10.365) (43.8532, -10.5181) knots 0 0 0 1 2 2 2
  spline S176 degree 2 poles (43.8532, -10.5181) (43.7247, -10.6737) (43.5815, -11.1455) (43.5815, -11.4394) knots 0 0 0 1 2 2 2
  spline S177 degree 2 poles (43.5815, -11.4394) (43.5815, -11.7531) (43.7322, -12.2051) (43.8631, -12.3607) knots 0 0 0 1 2 2 2
  spline S178 degree 2 poles (43.8631, -12.3607) (43.9915, -12.5114) (44.3348, -12.6646) (44.5275, -12.6646) knots 0 0 0 1 2 2 2
  spline S179 degree 2 poles (44.5275, -12.6646) (44.7029, -12.6646) (45.0017, -12.5781) (45.1178, -12.5139) knots 0 0 0 1 2 2 2
  spline S180 degree 2 poles (45.1178, -12.5139) (45.229, -12.4497) (45.3945, -12.3163) (45.4414, -12.2694) knots 0 0 0 1 2 2 2
  line L139 (45.4414, -12.2694) -> (45.471, -12.2694)
  line L140 (45.471, -12.2694) -> (45.471, -12.7535)
  spline S181 degree 2 poles (45.471, -12.7535) (45.3698, -12.8004) (45.1919, -12.8869) (45.066, -12.9264) knots 0 0 0 1 2 2 2
  spline S182 degree 2 poles (45.066, -12.9264) (44.9326, -12.9708) (44.7053, -13.0153) (44.5226, -13.0153) knots 0 0 0 1 2 2 2
  spline S183 degree 2 poles (47.0938, -12.7189) (47.0469, -12.7535) (46.8888, -12.877) (46.8147, -12.914) knots 0 0 0 1 2 2 2
  spline S184 degree 2 poles (46.8147, -12.914) (46.7135, -12.9684) (46.5233, -13.0252) (46.3504, -13.0252) knots 0 0 0 1 2 2 2
  spline S185 degree 2 poles (46.3504, -13.0252) (46.2096, -13.0252) (45.9552, -12.919) (45.8588, -12.8226) knots 0 0 0 1 2 2 2
  spline S186 degree 2 poles (45.8588, -12.8226) (45.7674, -12.7288) (45.6563, -12.4521) (45.6563, -12.299) knots 0 0 0 1 2 2 2
  spline S187 degree 2 poles (45.6563, -12.299) (45.6563, -12.0619) (45.8564, -11.726) (46.0737, -11.6296) knots 0 0 0 1 2 2 2
  spline S188 degree 2 poles (46.0737, -11.6296) (46.2664, -11.5407) (46.79, -11.474) (47.0938, -11.4567) knots 0 0 0 1 2 2 2
  line L141 (47.0938, -11.4567) -> (47.0938, -11.3826)
  spline S189 degree 2 poles (47.0938, -11.3826) (47.0938, -11.2492) (47.0123, -11.0838) (46.9382, -11.0368) knots 0 0 0 1 2 2 2
  spline S190 degree 2 poles (46.9382, -11.0368) (46.8641, -10.9899) (46.6517, -10.9602) (46.5381, -10.9602) knots 0 0 0 1 2 2 2
  spline S191 degree 2 poles (46.5381, -10.9602) (46.4047, -10.9602) (46.0441, -11.0393) (45.8638, -11.1159) knots 0 0 0 1 2 2 2
  line L142 (45.8638, -11.1159) -> (45.8415, -11.1159)
  line L143 (45.8415, -11.1159) -> (45.8415, -10.7231)
  spline S192 degree 2 poles (45.8415, -10.7231) (45.9478, -10.6935) (46.3454, -10.6194) (46.5406, -10.6194) knots 0 0 0 1 2 2 2
  spline S193 degree 2 poles (46.5406, -10.6194) (46.7777, -10.6194) (47.1013, -10.6935) (47.2297, -10.7898) knots 0 0 0 1 2 2 2
  spline S194 degree 2 poles (47.2297, -10.7898) (47.3557, -10.8837) (47.4792, -11.1826) (47.4792, -11.3974) knots 0 0 0 1 2 2 2
  line L144 (47.4792, -11.3974) -> (47.4792, -12.961)
  line L145 (47.4792, -12.961) -> (47.0938, -12.961)
  line L146 (47.0938, -12.961) -> (47.0938, -12.7189)
  line L147 (47.0938, -12.3978) -> (47.0938, -11.763)
  spline S195 degree 2 poles (47.0938, -11.763) (46.9555, -11.7754) (46.5381, -11.8173) (46.4072, -11.8569) knots 0 0 0 1 2 2 2
  spline S196 degree 2 poles (46.4072, -11.8569) (46.254, -11.9038) (46.054, -12.0989) (46.054, -12.2718) knots 0 0 0 1 2 2 2
  spline S197 degree 2 poles (46.054, -12.2718) (46.054, -12.4694) (46.2763, -12.6695) (46.4887, -12.6695) knots 0 0 0 1 2 2 2
  spline S198 degree 2 poles (46.4887, -12.6695) (46.669, -12.6695) (46.9654, -12.5139) (47.0938, -12.3978) knots 0 0 0 1 2 2 2
  spline S199 degree 2 poles (48.6376, -13.0153) (48.4079, -13.0153) (48.0102, -12.8918) (47.8793, -12.8226) knots 0 0 0 1 2 2 2
  line L148 (47.8793, -12.8226) -> (47.8793, -12.3904)
  line L149 (47.8793, -12.3904) -> (47.8991, -12.3904)
  spline S200 degree 2 poles (47.8991, -12.3904) (47.9485, -12.4299) (48.0818, -12.5238) (48.193, -12.5756) knots 0 0 0 1 2 2 2
  spline S201 degree 2 poles (48.193, -12.5756) (48.2893, -12.6226) (48.5265, -12.6917) (48.6524, -12.6917) knots 0 0 0 1 2 2 2
  spline S202 degree 2 poles (48.6524, -12.6917) (48.7438, -12.6917) (48.9538, -12.6497) (49.0032, -12.6152) knots 0 0 0 1 2 2 2
  spline S203 degree 2 poles (49.0032, -12.6152) (49.0748, -12.5682) (49.139, -12.462) (49.139, -12.3533) knots 0 0 0 1 2 2 2
  spline S204 degree 2 poles (49.139, -12.3533) (49.139, -12.2175) (48.9908, -12.0767) (48.8006, -12.0298) knots 0 0 0 1 2 2 2
  spline S205 degree 2 poles (48.8006, -12.0298) (48.7265, -12.0125) (48.4894, -11.9631) (48.3881, -11.9359) knots 0 0 0 1 2 2 2
  spline S206 degree 2 poles (48.3881, -11.9359) (48.1263, -11.8593) (47.8892, -11.5432) (47.8892, -11.3184) knots 0 0 0 1 2 2 2
  spline S207 degree 2 poles (47.8892, -11.3184) (47.8892, -11.0072) (48.356, -10.6194) (48.7413, -10.6194) knots 0 0 0 1 2 2 2
  spline S208 degree 2 poles (48.7413, -10.6194) (48.9315, -10.6194) (49.3169, -10.7132) (49.4478, -10.7849) knots 0 0 0 1 2 2 2
  line L150 (49.4478, -10.7849) -> (49.4478, -11.1974)
  line L151 (49.4478, -11.1974) -> (49.428, -11.1974)
  spline S209 degree 2 poles (49.428, -11.1974) (49.2798, -11.0788) (48.9192, -10.943) (48.7339, -10.943) knots 0 0 0 1 2 2 2
  spline S210 degree 2 poles (48.7339, -10.943) (48.5437, -10.943) (48.2819, -11.1035) (48.2819, -11.2641) knots 0 0 0 1 2 2 2
  spline S211 degree 2 poles (48.2819, -11.2641) (48.2819, -11.4098) (48.4375, -11.5506) (48.6104, -11.595) knots 0 0 0 1 2 2 2
  spline S212 degree 2 poles (48.6104, -11.595) (48.6944, -11.6173) (48.9068, -11.6617) (49.0229, -11.6889) knots 0 0 0 1 2 2 2
  spline S213 degree 2 poles (49.0229, -11.6889) (49.2749, -11.7531) (49.5317, -12.0471) (49.5317, -12.3015) knots 0 0 0 1 2 2 2
  spline S214 degree 2 poles (49.5317, -12.3015) (49.5317, -12.4497) (49.4157, -12.7115) (49.302, -12.8078) knots 0 0 0 1 2 2 2
  spline S215 degree 2 poles (49.302, -12.8078) (49.181, -12.9091) (48.8723, -13.0153) (48.6376, -13.0153) knots 0 0 0 1 2 2 2
  spline S216 degree 2 poles (50.8828, -13.0128) (50.3345, -13.0128) (49.7318, -12.3978) (49.7318, -11.8297) knots 0 0 0 1 2 2 2
  spline S217 degree 2 poles (49.7318, -11.8297) (49.7318, -11.2715) (50.3172, -10.6095) (50.789, -10.6095) knots 0 0 0 1 2 2 2
  spline S218 degree 2 poles (50.789, -10.6095) (51.0014, -10.6095) (51.3299, -10.733) (51.451, -10.8639) knots 0 0 0 1 2 2 2
  spline S219 degree 2 poles (51.451, -10.8639) (51.5745, -10.9948) (51.7054, -11.3727) (51.7054, -11.6469) knots 0 0 0 1 2 2 2
  line L152 (51.7054, -11.6469) -> (51.7054, -11.8569)
  line L153 (51.7054, -11.8569) -> (50.1221, -11.8569)
  spline S220 degree 2 poles (50.1221, -11.8569) (50.1221, -12.2545) (50.5222, -12.6769) (50.8779, -12.6769) knots 0 0 0 1 2 2 2
  spline S221 degree 2 poles (50.8779, -12.6769) (51.0039, -12.6769) (51.2484, -12.6201) (51.3472, -12.5756) knots 0 0 0 1 2 2 2
  spline S222 degree 2 poles (51.3472, -12.5756) (51.451, -12.5262) (51.5942, -12.4398) (51.6411, -12.4003) knots 0 0 0 1 2 2 2
  line L154 (51.6411, -12.4003) -> (51.6634, -12.4003)
  line L155 (51.6634, -12.4003) -> (51.6634, -12.8202)
  spline S223 degree 2 poles (51.6634, -12.8202) (51.5967, -12.8473) (51.3941, -12.9264) (51.3151, -12.9486) knots 0 0 0 1 2 2 2
  spline S224 degree 2 poles (51.3151, -12.9486) (51.204, -12.9807) (51.0212, -13.0128) (50.8828, -13.0128) knots 0 0 0 1 2 2 2
  spline S225 degree 2 poles (51.3299, -11.5629) (51.325, -11.4073) (51.2608, -11.1801) (51.199, -11.1035) knots 0 0 0 1 2 2 2
  spline S226 degree 2 poles (51.199, -11.1035) (51.1323, -11.0171) (50.9224, -10.9257) (50.7668, -10.9257) knots 0 0 0 1 2 2 2
  spline S227 degree 2 poles (50.7668, -10.9257) (50.6136, -10.9257) (50.3987, -11.0171) (50.3098, -11.106) knots 0 0 0 1 2 2 2
  spline S228 degree 2 poles (50.3098, -11.106) (50.2234, -11.1974) (50.1344, -11.4172) (50.1221, -11.5629) knots 0 0 0 1 2 2 2
  line L156 (50.1221, -11.5629) -> (51.3299, -11.5629)
  point P0 (39.6875, 0)
  constraints: 2 end point, 2 midpoint, 1 horizontal
extrude "Extrusion3" cut sketch "Sketch4" against normal blind 1.27
body "Solid1"
